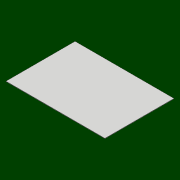
# Autodesk Inventor part: filecase
Saved by Autodesk Inventor 2018 (Build 220112000, 112)
## iProperties
Created: 2022-01-01
Part Number: filecase
Material: 一般
Document SubType Name: Modeling
Designer: gisen
Density: 1 g/cm^3
Appearance: 既定
Author: gisen
Autodesk Inventor part; units mm, degrees
ref_plane "YZ Plane" through (0, 0, 0) normal (1, 0, 0) x (0, 1, 0)
ref_plane "XZ Plane" through (0, 0, 0) normal (0, 1, 0) x (-1, 0, 0)
ref_plane "XY Plane" through (0, 0, 0) normal (0, 0, 1) x (1, 0, 0)
sketch "スケッチ1" plane through (0, 0, 0) normal (0, 0, 1) x (1, 0, 0)
  line L0 (-265, 185) -> (265, 185)
  line L1 (265, 185) -> (265, -185)
  line L2 (265, -185) -> (-265, -185)
  line L3 (-265, -185) -> (-265, 185)
  point P0 (0, 0)
  point P1 (0, 185)
  point P2 (-265, 0)
  dimension "d0" = 370
  dimension "d1" = 530
  constraints: 8 end point, 2 midpoint, 2 parallel, 1 horizontal, 1 horizontal alignment, 1 perpendicular, 1 vertical alignment
  measures "d0" distance of L2.end L0.start
  measures "d1" distance of L0.start L0.end
extrude "押し出し1" add sketch "スケッチ1" along normal blind 2
